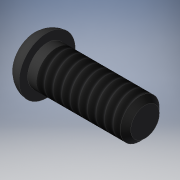
# Autodesk Inventor part: SNZS-M1.6-4
Saved by Autodesk Inventor 2019 (Build 230136000, 136)
## iProperties
Created: 2022-09-02
Part Number: SNZS-M1.6-4
Material: Generic
Catalog Web Link: www.cadenas.de
Description: SNZS-Pan Head Machine Screw for Precision Instruments
Vendor: NBK
Document SubType Name: Modeling
Designer: psAdmin
Manufacturer: NBK
Mass: 0.0094227 g
Surface Area: 0.329749 cm^2
Volume: 0.0094227 cm^3
Density: 1 g/cm^3
Appearance: PSOLRGB-175-175-175
Category: PARTsolutions
Company: NBK
Title: SNZS-M1.6-4
Author: Cadenas PARTsolutions
Comments: Pan Head Machine Screw for Precision Instruments
PSOL_IDENT_0: {$CADENAS_DATA/23d-libs/nbk/e_nedzi_com/miniature_screws/snzs.prj},161 {VTYP=3D},{NB=SNZS-M1.6-4},{L
PSOL_IDENT_1: INA=SNZS-M1.6-4},{NN=SNZS},{DATE=29.08.2022 00:26:45},{GEOMDATE=12.07.2022 05:41:24},{VERSION=},{LIN
PSOL_IDENT_2: EID=430},{WBVAR=},{WBNUMERIC=}  {NB=SNZS-M1.6-4},{LINA=SNZS-M1.6-4},{KT=DUMMY},{CN=SNZS-M1.6-4},{M=M
PSOL_IDENT_3: 1.6},{L=4.0},{D1=2.3},{L1=0.50},{A=0.00},{MT=0.100},{MASS=0.09},{NDM=1.6},{KDM=1.17},{VER=2}
NB: SNZS-M1.6-4
NN: SNZS
NT: Pan Head Machine Screw for Precision Instruments
NBSYN: $CN.
LINA: SNZS-M1.6-4
CATALOG: NBK (Nabeya Bi-tech Kaisha
CN: SNZS-M1.6-4
M: M1.6
L: 4
D1: 2.3
L1: 0.5
A: 0
SUPPLIER: NBK
ARTICLENO: SNZS-M1.6-4
BOMINFO: SNZS-M1.6-4
CREATOR: CADENAS GmbH
Autodesk Inventor part; units mm, degrees
ref_plane "YZ Plane" through (0, 0, 0) normal (1, 0, 0) x (0, 1, 0)
ref_plane "XZ Plane" through (0, 0, 0) normal (0, 1, 0) x (-1, 0, 0)
ref_plane "XY Plane" through (0, 0, 0) normal (0, 0, 1) x (1, 0, 0)
sketch "Sketch_1" plane through (0, 0, 0) normal (0, 0, 1) x (1, 0, 0)
  line L0 (4, 0) -> (-0.5, 0)
  line L1 (-0.5, 0) -> (-0.5, 0.92)
  arc A0 (0, 1.15) -> (-0.5, 0.92) centre (0.0416, 0.4012) ccw
  line L2 (0, 1.15) -> (0, 0.8)
  line L3 (0, 0.8) -> (3.7855, 0.8)
  line L4 (3.7855, 0.8) -> (4, 0.5855)
  line L5 (4, 0.5855) -> (4, 0)
  line L6 (4, 0) -> (-0.5, 0)
  constraints: 14 end point, 2 point on circle, 1 centre point
revolve "Revolution1" add sketch "Sketch_1" angle 360 about axis through (4, 0, 0) along (1, 0, 0)
thread "Thread1" size "M1.6x0.35" class "6g" standard "ISO Metric profile" length 3.4131
sketch "Sketch_2" plane through (0, 0, 0) normal (0, 0, 1) x (1, 0, 0)
  line L0 (-0.5, -0.69) -> (0.25, -0.345)
  line L1 (0.25, -0.345) -> (0.375, 0)
  line L2 (0.375, 0) -> (0.25, 0.345)
  line L3 (0.25, 0.345) -> (-0.5, 0.69)
  line L4 (-0.5, 0.69) -> (-0.5, -0.69)
  constraints: 10 end point
extrude "Extrusion1" cut sketch "Sketch_2" along normal mid plane 0.23
sketch "Sketch_3" plane through (0, 0, 0) normal (0, 1, 0) x (-1, 0, 0)
  line L0 (0.5, 0.69) -> (-0.25, 0.345)
  line L1 (-0.25, 0.345) -> (-0.375, 0)
  line L2 (-0.375, 0) -> (-0.25, -0.345)
  line L3 (-0.25, -0.345) -> (0.5, -0.69)
  line L4 (0.5, -0.69) -> (0.5, 0.69)
  constraints: 10 end point
extrude "Extrusion2" cut sketch "Sketch_3" along normal mid plane 0.23
body "Solid1"
